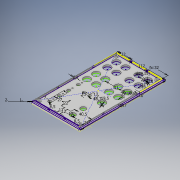
# Autodesk Inventor part: tapa2
Saved by Autodesk Inventor 2019 (Build 230136000, 136)
## iProperties
Created: 2020-09-11
Part Number: tapa2
Material: Generic
Document SubType Name: Modeling
Designer: assman
Density: 1 g/cm^3
Appearance: Default
Author: assman
## iProperties of the stored document tapa2_3DPrint.ipt
Created: 2020-09-11
Part Number: tapa2_3DPrint
Material: Generic
Document SubType Name: Modeling
Designer: assman
Density: 1 g/cm^3
Appearance: Default
Author: assman
Autodesk Inventor part; units mm, degrees
ref_plane "YZ Plane" through (0, 0, 0) normal (1, 0, 0) x (0, 1, 0)
ref_plane "XZ Plane" through (0, 0, 0) normal (0, 1, 0) x (-1, 0, 0)
ref_plane "XY Plane" through (0, 0, 0) normal (0, 0, 1) x (1, 0, 0)
sketch "Sketch1" plane through (0, 0, 0) normal (0, 1, 0) x (-1, 0, 0)
  line L0 (54, 98.5) -> (-54, 98.5)
  line L1 (-56, 96.5) -> (-56, -96.5)
  line L2 (-54, -98.5) -> (54, -98.5)
  line L3 (56, -96.5) -> (56, 96.5)
  line L4 (56, 98.5) -> (-56, -98.5) construction
  line L5 (-56, 98.5) -> (56, -98.5) construction
  line L6 (52, 95.5) -> (-52, 95.5)
  line L7 (-53, 94.5) -> (-53, -94.5)
  line L8 (-52, -95.5) -> (52, -95.5)
  line L9 (53, -94.5) -> (53, 94.5)
  arc A0 (56, 96.5) -> (54, 98.5) centre (54, 96.5) ccw
  arc A1 (-54, 98.5) -> (-56, 96.5) centre (-54, 96.5) ccw
  arc A2 (54, -98.5) -> (56, -96.5) centre (54, -96.5) ccw
  arc A3 (-56, -96.5) -> (-54, -98.5) centre (-54, -96.5) ccw
  line L10 (50.7, 94.2) -> (-50.7, 94.2)
  line L11 (-51.7, 93.2) -> (-51.7, -93.2)
  line L12 (-50.7, -94.2) -> (50.7, -94.2)
  line L13 (51.7, -93.2) -> (51.7, 93.2)
  arc A4 (53, 94.5) -> (52, 95.5) centre (52, 94.5) ccw
  arc A5 (51.7, 93.2) -> (50.7, 94.2) centre (50.7, 93.2) ccw
  arc A6 (52, -95.5) -> (53, -94.5) centre (52, -94.5) ccw
  arc A7 (50.7, -94.2) -> (51.7, -93.2) centre (50.7, -93.2) ccw
  arc A8 (-53, -94.5) -> (-52, -95.5) centre (-52, -94.5) ccw
  arc A9 (-51.7, -93.2) -> (-50.7, -94.2) centre (-50.7, -93.2) ccw
  arc A10 (-52, 95.5) -> (-53, 94.5) centre (-52, 94.5) ccw
  arc A11 (-50.7, 94.2) -> (-51.7, 93.2) centre (-50.7, 93.2) ccw
  point P0 (0, 0)
  dimension "d0" = 112
  dimension "d1" = 197
  dimension "d2" = 3
  dimension "d3" = 2
  dimension "d4" = 1.3
  dimension "d7" = 1
  constraints: 28 end point, 24 point on circle, 24 tangent, 12 centre point, 10 equal radius, 8 point on line, 6 parallel, 3 perpendicular, 2 midpoint, 1 horizontal, 6 other
  measures "d0" distance of L5.end L4.end
  measures "d1" distance of L4.end L5.start
  measures "d2" distance between parallel lines of L3 L9
  measures "d3" radius of A0
  measures "d4" distance between parallel lines of L9 L13
  measures "d7" radius of A4
extrude "Extrusion1" add sketch "Sketch1" against normal blind 4 contours A0 L3 A2 L2 A3 L1 A1 L0 | A4 L9 A6 L8 A8 L7 A10 L6 | A5 L13 A7 L12 A9 L11 A11 L10
extrude "Extrusion2" add sketch "Sketch1" along normal blind 3 contours A4 L9 A6 L8 A8 L7 A10 L6
sketch "Sketch2" plane through (0, 3, 0) normal (0, 1, 0) x (1, 0, 0)
  line L0 (-52.9091, -43.5) -> (-51.6091, -43.5)
  line L1 (-51.6091, -43.5) -> (-51.6091, -38.5)
  line L2 (-51.6091, -38.5) -> (-52.9091, -38.5)
  line L3 (-52.9091, -38.5) -> (-52.9091, -43.5)
  line L4 (-52, -95.5) -> (52, -95.5) projected
  line L5 (52, -43.5) -> (53.3, -43.5)
  line L6 (53.3, -43.5) -> (53.3, -38.5)
  line L7 (53.3, -38.5) -> (52, -38.5)
  line L8 (52, -38.5) -> (52, -43.5)
  line L9 (-53, -94.5) -> (-53, 94.5) projected
  line L10 (-53, 38.5) -> (-51.7, 38.5)
  line L11 (-51.7, 38.5) -> (-51.7, 43.5)
  line L12 (-51.7, 43.5) -> (-53, 43.5)
  line L13 (-53, 43.5) -> (-53, 38.5)
  line L14 (52, 95.5) -> (-52, 95.5) projected
  line L15 (51.7, -93.2) -> (51.7, 93.2) projected
  line L16 (53, 94.5) -> (53, -94.5) projected
  line L17 (51.7, 43.5) -> (53, 43.5)
  line L18 (53, 43.5) -> (53, 38.5)
  line L19 (53, 38.5) -> (51.7, 38.5)
  line L20 (51.7, 38.5) -> (51.7, 43.5)
  point P0 (0, 0)
  dimension "d10" = 1.3
  dimension "d11" = 5
  dimension "d12" = 52
  dimension "d13" = 1.3
  dimension "d14" = 1.3
  dimension "d15" = 5
  dimension "d16" = 52
  constraints: 32 end point, 8 parallel, 4 horizontal, 4 perpendicular, 3 point on line
  measures "d10" distance of L2.end L1.end
  measures "d11" distance of L1.end L0.end
  measures "d12" distance between parallel lines of L4 L0
  measures "d13" distance of L7.end L6.end
  measures "d14" distance of L12.end L11.end
  measures "d15" distance of L11.end L10.end
  measures "d16" distance between parallel lines of L14 L12
extrude "Extrusion3" cut sketch "Sketch2" against normal blind 3
sketch "Sketch3" plane through (0, 0, 0) normal (0, 1, 0) x (1, 0, 0)
  circle A0 centre (-47, -89) radius 3.5
  line L0 (-54, -98.5) -> (54, -98.5) projected
  line L1 (-56, 96.5) -> (-56, -96.5) projected
  circle A1 centre (-47, 89) radius 3.5
  circle A2 centre (47, -89) radius 3.5
  circle A3 centre (47, 89) radius 3.5
  line L2 (56, -96.5) -> (56, 96.5) projected
  line L3 (54, 98.5) -> (-54, 98.5) projected
  point P0 (0, 0)
  dimension "d19" = 7
  dimension "d20" = 9.5
  dimension "d21" = 9
  dimension "d22" = 7
  dimension "d23" = 7
  dimension "d24" = 7
  dimension "d25" = 9.5
  dimension "d26" = 9
  dimension "d27" = 9.5
  dimension "d28" = 9
  dimension "d29" = 9.5
  dimension "d30" = 9
  constraints: 4 centre point
  measures "d19" diameter of A0
  measures "d20" distance from line of L0 A0.centre
  measures "d21" distance from line of L1 A0.centre
  measures "d22" diameter of A1
  measures "d23" diameter of A2
  measures "d24" diameter of A3
  measures "d25" distance from line of L0 A2.centre
  measures "d26" distance from line of L2 A2.centre
  measures "d27" distance from line of L3 A3.centre
  measures "d28" distance from line of L2 A3.centre
  measures "d29" distance from line of L3 A1.centre
  measures "d30" distance from line of L1 A1.centre
extrude "Extrusion4" add sketch "Sketch3" along normal blind 2.8
sketch "Sketch5" plane through (0, -4, 0) normal (0, -1, 0) x (1, 0, 0)
  circle A0 centre (47, 89) radius 3.5 projected
  circle A1 centre (47, -89) radius 3.5 projected
  circle A2 centre (-47, -89) radius 3.5 projected
  circle A3 centre (-47, 89) radius 3.5 projected
  point P0 (0, 0)
  constraints: 4 coincident
hole "Hole1" at (47, -4, 89) at (47, -4, -89) at (-47, -4, -89) at (-47, -4, 89) direction (0, 1, 0) diameter 3 end through all counterbore diameter 6 counterbore depth 2
sketch "Sketch7" plane through (0, -4, 0) normal (0, -1, 0) x (1, 0, 0)
  circle A0 centre (-47, -89) radius 3 construction
  circle A1 centre (47, 89) radius 3 construction
  circle A2 centre (47, -89) radius 3 construction
  circle A3 centre (-47, 89) radius 3 construction
  line L0 (54, 98.5) -> (-54, 98.5) construction
  arc A4 (-54, 98.5) -> (-56, 96.5) centre (-54, 96.5) ccw construction
  line L1 (-56, 96.5) -> (-56, -96.5) construction
  arc A5 (-56, -96.5) -> (-54, -98.5) centre (-54, -96.5) ccw construction
  line L2 (-54, -98.5) -> (54, -98.5) construction
  arc A6 (54, -98.5) -> (56, -96.5) centre (54, -96.5) ccw construction
  line L3 (56, -96.5) -> (56, 96.5) construction
  arc A7 (56, 96.5) -> (54, 98.5) centre (54, 96.5) ccw construction
  line L4 (46, 88.5) -> (46, -88.5) construction
  line L5 (46, -88.5) -> (-46, -88.5) construction
  line L6 (-46, -88.5) -> (-46, 88.5) construction
  line L7 (-46, 88.5) -> (46, 88.5) construction
  circle A8 centre (36, -78.5) radius 7.85
  circle A9 centre (36, -78.5) radius 9.575 construction
  line L8 (46, 84.9773) -> (5.5, 84.9773) construction
  line L9 (5.5, 84.9773) -> (5.5, 67.9773) construction
  line L10 (5.5, 67.9773) -> (46, 67.9773) construction
  line L11 (46, 67.9773) -> (46, 84.9773) construction
  circle A10 centre (18.5, 76.4773) radius 6
  line L12 (46, 60.9773) -> (5.5, 60.9773) construction
  line L13 (5.5, 60.9773) -> (5.5, 43.9773) construction
  line L14 (5.5, 43.9773) -> (46, 43.9773) construction
  circle A11 centre (18.5, 52.4773) radius 6
  line L15 (-43.986, 84.9838) -> (-16.986, 84.9838) construction
  line L16 (-16.986, 84.9838) -> (-16.986, 67.9838) construction
  line L17 (-16.986, 67.9838) -> (-43.986, 67.9838) construction
  line L18 (-43.986, 67.9838) -> (-43.986, 84.9838) construction
  circle A12 centre (-34.986, 76.4838) radius 3.5
  line L19 (-16.986, 45.9838) -> (-43.986, 45.9838) construction
  line L20 (-43.986, 45.9838) -> (-43.986, 62.9838) construction
  line L21 (-16.986, 62.9838) -> (-16.986, 45.9838) construction
  circle A13 centre (-34.986, 54.4838) radius 3.5
  line L22 (-16.986, 23.9838) -> (-43.986, 23.9838) construction
  line L23 (-43.986, 23.9838) -> (-43.986, 40.9838) construction
  line L24 (-16.986, 40.9838) -> (-16.986, 23.9838) construction
  circle A14 centre (-34.986, 32.4838) radius 3.5
  line L25 (-16.986, 1.9838) -> (-43.986, 1.9838) construction
  line L26 (-43.986, 1.9838) -> (-43.986, 18.9838) construction
  line L27 (-16.986, 18.9838) -> (-16.986, 1.9838) construction
  circle A15 centre (-34.986, 10.4838) radius 3.5
  line L28 (-34.986, 76.4838) -> (65.1824, 76.4838) construction
  circle A16 centre (0, 18.9519) radius 3
  line L29 (6.5, 25.4519) -> (-6.5, 25.4519) construction
  line L30 (-6.5, 25.4519) -> (-6.5, 12.4519) construction
  line L31 (-6.5, 12.4519) -> (6.5, 12.4519) construction
  line L32 (6.5, 12.4519) -> (6.5, 25.4519) construction
  line L33 (6.5, 25.4519) -> (-6.5, 12.4519) construction
  line L34 (-6.5, 25.4519) -> (6.5, 12.4519) construction
  circle A17 centre (36, -57.5) radius 7.85
  circle A18 centre (36, -57.5) radius 9.575 construction
  circle A19 centre (15, -78.5) radius 7.85
  circle A20 centre (15, -78.5) radius 9.575 construction
  circle A21 centre (15, -57.5) radius 7.85
  circle A22 centre (15, -57.5) radius 9.575 construction
  circle A23 centre (36, -31.8) radius 7.85
  circle A24 centre (36, -31.8) radius 9.575 construction
  circle A25 centre (36, -10.8) radius 7.85
  circle A26 centre (36, -10.8) radius 9.575 construction
  circle A27 centre (15, -31.8) radius 7.85
  circle A28 centre (15, -31.8) radius 9.575 construction
  circle A29 centre (15, -10.8) radius 7.85
  circle A30 centre (15, -10.8) radius 9.575 construction
  circle A31 centre (-15, -31.8) radius 7.85
  circle A32 centre (-15, -31.8) radius 9.575 construction
  circle A33 centre (-36, -31.8) radius 9.575 construction
  circle A34 centre (-36, -31.8) radius 7.85
  circle A35 centre (-36, -10.8) radius 9.575 construction
  circle A36 centre (-36, -10.8) radius 7.85
  circle A37 centre (-15, -10.8) radius 7.85
  circle A38 centre (-15, -10.8) radius 9.575 construction
  circle A39 centre (-15, -57.5) radius 7.85
  circle A40 centre (-15, -57.5) radius 9.575 construction
  circle A41 centre (-36, -57.5) radius 9.575 construction
  circle A42 centre (-36, -57.5) radius 7.85
  circle A43 centre (-36, -78.5) radius 9.575 construction
  circle A44 centre (-36, -78.5) radius 7.85
  circle A45 centre (-15, -78.5) radius 7.85
  circle A46 centre (-15, -78.5) radius 9.575 construction
  circle A47 centre (28.15, 18.9519) radius 7.85
  circle A48 centre (28.15, 18.9519) radius 9.75 construction
  point P0 (0, 0)
  point P1 (46, 76.4773)
  dimension "d40" = 10
  dimension "d41" = 15.7
  dimension "d42" = 10
  dimension "d43" = 10
  dimension "d44" = 19.15
  dimension "d53" = 40.5
  dimension "d54" = 17
  dimension "d55" = 12
  dimension "d56" = 13
  dimension "d57" = 8.5
  dimension "d60" = 24
  dimension "d65" = 27
  dimension "d66" = 17
  dimension "d67" = 7
  dimension "d68" = 9
  dimension "d69" = 8.5
  dimension "d72" = 22
  dimension "d77" = 6
  dimension "d78" = 13
  dimension "d79" = 13
  dimension "d82" = 21
  dimension "d85" = 21
  dimension "d88" = 15.7
  dimension "d89" = 19.15
  dimension "d90" = 10
  dimension "d93" = 21
  dimension "d96" = 21
  dimension "d101" = 51
  dimension "d106" = 15.7
  dimension "d107" = 19.5
  constraints: 62 end point, 41 centre point, 17 coincident, 7 horizontal, 6 parallel, 4 vertical, 3 midpoint, 3 perpendicular, 1 point on line, 95 other
  measures "d40" distance between parallel lines of L3 L4
  measures "d41" diameter of A8
  measures "d42" distance from line of L5 A8.centre
  measures "d43" distance from line of L4 A8.centre
  measures "d44" diameter of A9
  measures "d53" distance of L10.end L9.end
  measures "d54" distance of L9.end L8.end
  measures "d55" diameter of A10
  measures "d56" distance from line of L9 A10.centre
  measures "d57" distance from line of L8 A10.centre
  measures "d60" distance of L8.start L12.start
  measures "d65" distance of L16.end L17.end
  measures "d66" distance of L15.end L16.end
  measures "d67" diameter of A12
  measures "d68" distance from line of L18 L28.start
  measures "d69" distance from line of L15 L28.start
  measures "d72" distance of L16.end L19.start
  measures "d77" diameter of A16
  measures "d78" distance of L31.end L30.end
  measures "d79" distance of L30.end L29.end
  measures "d82" distance of A8.centre A17.centre
  measures "d85" distance of A8.centre A19.centre
  measures "d88" diameter of A23
  measures "d89" diameter of A24
  measures "d93" distance of A23.centre A25.centre
  measures "d96" distance of A23.centre A27.centre
  measures "d101" distance of A23.centre A31.centre
  measures "d106" diameter of A47
  measures "d107" diameter of A48
extrude "Extrusion5" cut sketch "Sketch7" against normal through all
sketch "Sketch8" plane through (0, 0, 0) normal (0, 1, 0) x (1, 0, 0)
  line L0 (-16.986, -67.9838) -> (-43.986, -67.9838) construction
  line L1 (-16.986, -45.9838) -> (-43.986, -45.9838) construction
  line L2 (-16.986, -23.9838) -> (-43.986, -23.9838) construction
  line L3 (-16.986, -1.9838) -> (-43.986, -1.9838) construction
  line L4 (6.5, -12.4519) -> (6.5, -25.4519) construction
  point P0 (0, 0)
  point P1 (-34.9799, -67.9838)
  point P2 (-34.9799, -45.9838)
  point P3 (-34.9799, -23.9838)
  point P4 (-34.9799, -1.9838)
  constraints: 4 point on line
hole "Hole2" at (-34.9799, 0, 23.9838) at (-34.9799, 0, 45.9838) at (-34.9799, 0, 67.9838) at (-34.9799, 0, 1.9838) direction (0, -1, 0) diameter 3 depth 2.4
sketch "Sketch9" plane through (0, 0, 0) normal (0, 1, 0) x (1, 0, 0)
  line L0 (0, -18.9519) -> (24, -18.9519) construction
  line L1 (0, -18.9519) -> (-17.45, -18.9519) construction
  circle A0 centre (0, -18.9519) radius 3 construction
  point P0 (0, 0)
  point P1 (12, -18.9519)
  point P2 (-12, -18.9519)
  dimension "d117" = 12
  dimension "d118" = 12
  constraints: 4 end point, 2 horizontal, 1 coincident, 1 midpoint, 1 point on line
  measures "d117" distance of L0.start point (12, -18.952)
  measures "d118" distance of L0.start point (-12, -18.952)
hole "Hole3" at (12, 0, 18.9519) at (-12, 0, 18.9519) direction (0, -1, 0) diameter 5 end through all
sketch "Sketch10" plane through (0, 3, 0) normal (0, 1, 0) x (1, 0, 0)
  line L0 (-52, 95.5) -> (52, 95.5) projected
  line L1 (50.7, 94.2) -> (-50.7, 94.2) projected
  line L2 (-21, 95.5) -> (-16, 95.5)
  line L3 (-16, 95.5) -> (-16, 94.2)
  line L4 (-16, 94.2) -> (-21, 94.2)
  line L5 (-21, 94.2) -> (-21, 95.5)
  line L6 (-53, 94.5) -> (-53, 43.5) projected
  line L7 (16, 95.5) -> (21, 95.5)
  line L8 (21, 95.5) -> (21, 94.2)
  line L9 (21, 94.2) -> (16, 94.2)
  line L10 (16, 94.2) -> (16, 95.5)
  line L11 (53, 43.5) -> (53, 94.5) projected
  line L12 (0, 0) -> (30.4979, 0) construction
  line L13 (-52, -95.5) -> (52, -95.5)
  line L14 (50.7, -94.2) -> (-50.7, -94.2)
  line L15 (-21, -95.5) -> (-16, -95.5)
  line L16 (-16, -95.5) -> (-16, -94.2)
  line L17 (-16, -94.2) -> (-21, -94.2)
  line L18 (-21, -94.2) -> (-21, -95.5)
  line L19 (21, -95.5) -> (21, -94.2)
  line L20 (16, -94.2) -> (16, -95.5)
  line L21 (16, -95.5) -> (21, -95.5)
  line L22 (52, -95.5) -> (-52, -95.5) projected
  line L23 (16, -94.2) -> (21, -94.2)
  line L24 (-21, -95.5) -> (-16, -95.5)
  line L25 (-16, -95.5) -> (-16, -94.2)
  line L26 (-16, -94.2) -> (-21, -94.2)
  line L27 (-21, -94.2) -> (-21, -95.5)
  line L28 (16, -95.5) -> (21, -95.5)
  line L29 (21, -95.5) -> (21, -94.2)
  line L30 (21, -94.2) -> (16, -94.2)
  line L31 (16, -94.2) -> (16, -95.5)
  dimension "d126" = 5
  dimension "d127" = 32
  dimension "d128" = 5
  dimension "d129" = 32
  constraints: 54 end point, 12 symmetric about line, 8 parallel, 8 point on line, 5 horizontal, 4 perpendicular
  measures "d126" distance of L3.end L4.end
  measures "d127" distance between parallel lines of L6 L5
  measures "d128" distance of L8.end L9.end
  measures "d129" distance between parallel lines of L8 L11
extrude "Extrusion6" cut sketch "Sketch10" against normal up to surface (3 mm away) contours L0 L3 L1 L5 | L0 L8 L1 L10
extrude "Extrusion7" cut sketch "Sketch10" against normal up to surface (3 mm away) contours L18 L14 L16 L13 | L20 L14 L19 L13
equation "\"d16\" = d12"
equation "\"d25\" = d20"
equation "\"d26\" = d21"
equation "\"d27\" = d25"
equation "\"d28\" = d26"
equation "\"d29\" = d27"
equation "\"d30\" = d21"
body "Solid1"
